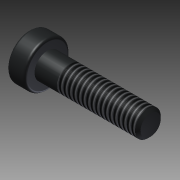
# Autodesk Inventor part: DIN-6912 - M4x16(F)
Saved by Autodesk Inventor 2011 SP1 (Build 150282100, 282)
## iProperties
Created: 2018-05-28
Part Number: DIN-6912 - M4x16(F)
Catalog Web Link: www.cadenas.de
Description: DIN-6912-Hexagon socket head cap screw with centre hole and low head
Vendor: FESTO
Document SubType Name: Modeling
Designer: psAdmin
Manufacturer: FESTO
Mass: 0.286347 g
Surface Area: 3.54698 cm^2
Volume: 0.286347 cm^3
Density: 1 g/cm^3
Category: PARTsolutions
Company: FESTO
Title: DIN-6912 - M4x16(F)
Author: Cadenas PARTsolutions
Comments: Hexagon socket head cap screw with centre hole and low head
PSOL_IDENT_0: {$CADENAS_DATA\23d-libs\festo\zyl_zubeh\din_6912\din_6912.prj},182 {VTYP=3D},{NB=DIN-6912 - M4x16(F)
PSOL_IDENT_1: },{LINA=DIN-6912 - M4x16(F)},{NN=DIN-6912},{DATE=16.11.2017 11:29:57},{GEOMDATE=16.11.2017 11:29:44}
PSOL_IDENT_2: ,{VERSION=},{LINEID=30},{LINESUBID=-1},{WBVAR=}  {NB=DIN-6912 - M4x16(F)},{LINA=DIN-6912 - M4x16(F)}
PSOL_IDENT_3: ,{KT=L},{IDNR=},{NENN=M4x16},{D=4.000},{L=16.000},{DK=3.141},{LS=1.400},{LG=3.500},{DK1=7.000},{DH=2
PSOL_IDENT_4: .000},{K=2.800},{R=0.200},{V=0.400},{S=3.000},{T1=1.600},{T2=3.300},{F=0.600},{DA=4.700},{DW=6.200}
NN: DIN-6912
NT: Hexagon socket head cap screw with centre hole and low head
NB: DIN-6912 - M4x16(F)
NBSYN: DIN-6912 - $NENN.(F)
LINA: DIN-6912 - M4x16(F)
ROWDESC: M4x16
D: 4.000
L: 16.000
DK: 3.141
LS: 1.400
LG: 3.500
DK1: 7.000
DH: 2.000
K: 2.800
R: 0.200
V: 0.400
S: 3.000
T1: 1.600
T2: 3.300
F: 0.600
DA: 4.700
DW: 6.200
SUPPLIER: FESTO
ARTICLENO: DIN-6912 - M4x16(F)
BOMINFO: DIN-6912 - M4x16(F)
CREATOR: CADENAS GmbH
Autodesk Inventor part; units mm, degrees
sketch "Sketch_1" plane through (0, 0, 0) normal (0, 0, 1) x (1, 0, 0)
  line L0 (16, 0) -> (1.5, 0)
  line L1 (1.5, 0) -> (0.5, 1)
  line L2 (0.5, 1) -> (-0.7, 1)
  line L3 (-0.7, 1) -> (-1.2, 1.5)
  line L4 (-1.2, 1.5) -> (-2.5679, 1.5)
  line L5 (-2.5679, 1.5) -> (-2.8, 1.7321)
  line L6 (-2.8, 1.7321) -> (-2.8, 3.1)
  arc A0 (-2.4, 3.5) -> (-2.8, 3.1) centre (-2.4, 3.1) ccw
  line L7 (-2.4, 3.5) -> (-0.4, 3.5)
  arc A1 (0, 3.1) -> (-0.4, 3.5) centre (-0.4, 3.1) ccw
  line L8 (0, 3.1) -> (0, 2)
  line L9 (0, 2) -> (15.5705, 2)
  line L10 (15.5705, 2) -> (16, 1.5705)
  line L11 (16, 1.5705) -> (16, 0)
  line L12 (16, 0) -> (1.5, 0)
  constraints: 26 end point, 4 point on circle, 2 centre point
revolve "Revolution1" add sketch "Sketch_1" angle 360 about axis through (16, 0, 0) along (-1, 0, 0)
thread "Thread1" size "M4x0.7" class "6g" standard "ISO Metric profile" length 12.0705
sketch "Sketch_2" plane through (-2.8, 0, 0) normal (1, 0, 0) x (0, 0, -1)
  line L0 (-1.5, -0.866) -> (0, -1.7321)
  line L1 (0, -1.7321) -> (1.5, -0.866)
  line L2 (1.5, -0.866) -> (1.5, 0.866)
  line L3 (1.5, 0.866) -> (0, 1.7321)
  line L4 (0, 1.7321) -> (-1.5, 0.866)
  line L5 (-1.5, 0.866) -> (-1.5, -0.866)
  constraints: 12 end point
extrude "Extrusion1" cut sketch "Sketch_2" along normal blind 1.6
ref_plane "MONTAGE_XY" through (0, 0, 0) normal (1, 0, 0) x (0, 0, -1)
ref_plane "MONTAGE_YZ" through (0, 0, 0) normal (0, 0, -1) x (0, 1, 0)
ref_plane "MONTAGE_ZX" through (0, 0, 0) normal (0, 1, 0) x (1, 0, 0)
ref_plane "Schrauben_punkt_XY" through (16, 0, 0) normal (-1, 0, 0) x (0, 0, -1)
ref_plane "Schrauben_punkt_YZ" through (16, 0, 0) normal (0, 0, -1) x (0, -1, 0)
ref_plane "Schrauben_punkt_ZX" through (16, 0, 0) normal (0, -1, 0) x (-1, 0, 0)
body "Solid1"
